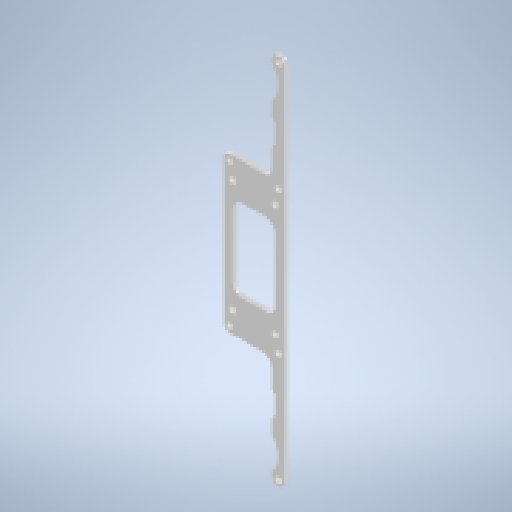
# Autodesk Inventor part: new_ude
Saved by Autodesk Inventor 2024 (Build 280153000, 153)
## iProperties
Created: 2023-12-16
Part Number: new_ude
Material: アルミニウム 2014-T4
Document SubType Name: Modeling
Designer: right
Density: 2.8 g/cm^3
Appearance: サテン
Mass: 3.58939 g
Surface Area: 23.5034 cm^2
Volume: 1.28192 cm^3
Author: right
Autodesk Inventor part; units mm, degrees
ref_plane "YZ Plane" through (0, 0, 0) normal (1, 0, 0) x (0, 1, 0)
ref_plane "XZ Plane" through (0, 0, 0) normal (0, 1, 0) x (-1, 0, 0)
ref_plane "XY Plane" through (0, 0, 0) normal (0, 0, 1) x (1, 0, 0)
sketch "スケッチ1" plane through (0, 0, 0) normal (0, 0, 1) x (1, 0, 0)
  circle A0 centre (-5.2771, -42.7168) radius 0.85 projected
  circle A1 centre (-21.2771, -42.7168) radius 0.85 projected
  circle A2 centre (-5.2771, -6.7168) radius 0.85 projected
  circle A3 centre (-13.2771, -13.2168) radius 8 projected
  line L0 (-3.2771, -4.7168) -> (-7.2771, -4.7168)
  line L1 (-7.2771, -4.7168) -> (-7.2771, -44.7168)
  line L2 (-7.2771, -44.7168) -> (-3.2771, -44.7168)
  line L3 (-3.2771, -44.7168) -> (-3.2771, -4.7168)
  line L4 (-3.2771, -44.7168) -> (-23.2771, -44.7168)
  line L5 (-23.2771, -44.7168) -> (-23.2771, -40.7168)
  line L6 (-23.2771, -40.7168) -> (-3.2771, -40.7168)
  line L7 (-3.2771, -40.7168) -> (-3.2771, -44.7168)
  circle A4 centre (-5.2771, -6.7168) radius 2
  circle A5 centre (-21.2771, -42.7168) radius 2
  circle A6 centre (-5.2771, -6.7168) radius 1.1
  circle A7 centre (-5.2771, -42.7168) radius 1.1
  circle A8 centre (-21.2771, -42.7168) radius 1.1
  line L8 (-5.2771, -66.2168) -> (-21.2771, -66.2168) construction
  circle A9 centre (-5.2771, -89.7168) radius 0.85
  circle A10 centre (-21.2771, -89.7168) radius 0.85
  circle A11 centre (-5.2771, -125.7168) radius 0.85
  circle A12 centre (-13.2771, -119.2168) radius 8
  line L9 (-3.2771, -127.7168) -> (-7.2771, -127.7168)
  line L10 (-7.2771, -127.7168) -> (-7.2771, -87.7168)
  line L11 (-7.2771, -87.7168) -> (-3.2771, -87.7168)
  line L12 (-3.2771, -87.7168) -> (-3.2771, -127.7168)
  line L13 (-3.2771, -87.7168) -> (-23.2771, -87.7168)
  line L14 (-23.2771, -87.7168) -> (-23.2771, -91.7168)
  line L15 (-23.2771, -91.7168) -> (-3.2771, -91.7168)
  line L16 (-3.2771, -91.7168) -> (-3.2771, -87.7168)
  circle A13 centre (-5.2771, -125.7168) radius 2
  circle A14 centre (-21.2771, -89.7168) radius 2
  circle A15 centre (-5.2771, -125.7168) radius 1.1
  circle A16 centre (-5.2771, -89.7168) radius 1.1
  circle A17 centre (-21.2771, -89.7168) radius 1.1
  line L17 (-3.2771, -44.7168) -> (-3.2771, -87.7168)
  line L18 (-23.2771, -44.7168) -> (-23.2771, -87.7168)
  line L19 (-6.4151, -24.526) -> (-6.4151, -30.526)
  line L20 (-6.2865, -24.2474) -> (-6.2865, -30.6046)
  line L21 (-6.2865, -30.6046) -> (-10.1437, -30.6046)
  line L22 (-10.1437, -24.2474) -> (-6.2865, -24.2474)
  line L23 (-6.4151, -107.9075) -> (-6.4151, -101.9075)
  line L24 (-6.2865, -108.1861) -> (-6.2865, -101.8289)
  line L25 (-6.2865, -101.8289) -> (-10.1437, -101.8289)
  line L26 (-10.1437, -108.1861) -> (-6.2865, -108.1861)
  line L27 (7.0429, 25.428) -> (7.0429, 23.728)
  point P0 (0, 0)
  point P1 (-3.2771, -42.7168)
  point P2 (-5.2771, -4.7168)
  point P3 (-13.2771, -44.7168)
  point P4 (-13.2771, -66.2168)
  point P5 (-3.2771, -89.7168)
  point P6 (-5.2771, -127.7168)
  point P7 (-13.2771, -87.7168)
  point P8 (-7.2771, -6.7168)
  point P9 (-7.2771, -7.9253)
  point P10 (-7.2771, -18.5083)
  point P11 (-7.2771, -40.7168)
  point P12 (-21.2771, -40.7168)
  point P13 (-23.2771, -42.7168)
  point P14 (-23.2771, -89.7168)
  point P15 (-21.2771, -91.7168)
  point P16 (-7.2771, -91.7168)
  point P17 (-7.2771, -113.9253)
  point P18 (-7.2771, -124.5083)
  point P19 (-7.2771, -125.7168)
  point P20 (-3.2771, -125.7168)
  point P21 (-3.2771, -6.7168)
  point P22 (-7.2771, -24.2474)
  point P23 (-7.2771, -30.6046)
  point P24 (-7.2771, -101.8289)
  point P25 (-7.2771, -108.1861)
  point P26 (7.0429, 24.578)
  dimension "d0" = 4
  dimension "d1" = 4
  dimension "d2" = 2.2
  dimension "d3" = 2.2
  dimension "d4" = 2.2
  dimension "d11" = 53
  constraints: 56 end point, 25 symmetric about line, 14 centre point, 10 coincident, 5 horizontal, 5 midpoint, 5 vertical, 4 parallel, 4 tangent, 2 perpendicular, 2 vertical alignment, 1 horizontal alignment, 17 other
  measures "d0" distance between parallel lines of L3 L1
  measures "d1" diameter of A5
  measures "d2" diameter of A6
  measures "d3" diameter of A7
  measures "d4" diameter of A8
  measures "d11" distance from line of A3.centre L8
extrude "押し出し1" add sketch "スケッチ1" along normal blind 1.5 contours A3 L1 A4 L3 L6 L21 L20 L22 | A4 | L3 L2 L1 L6 | L1 L4 A5 L6 | L17 L11 L13 L18 L4 L2 | A5 | L12 L15 L10 L11 | L4 L5 A5 | L10 L15 A14 L13 | L12 A13 L10 A12 L26 L24 L25 L15 | A14 L14 L13 | A14 | A13
fillet "フィレット1" radius 2 4 edges at (-7.2771, -108.1861, 0.75) (-7.2771, -101.8289, 0.75) (-7.2771, -24.2474, 0.75) (-7.2771, -30.6046, 0.75)
fillet "フィレット2" radius 2 4 edges at (-7.2771, -18.5083, 0.75) (-7.2771, -7.9253, 0.75) (-7.2771, -124.5083, 0.75) (-7.2771, -113.9253, 0.75)
fillet "フィレット3" radius 3 2 edges at (-7.2771, -91.7168, 0.75) (-7.2771, -40.7168, 0.75)
sketch "スケッチ2" plane through (0, 0, 1.5) normal (0, 0, 1) x (1, 0, 0)
  circle A0 centre (-6.2771, -47.7168) radius 1.1
  line L0 (-3.2771, -125.7168) -> (-3.2771, -6.7168) projected
  circle A1 centre (-5.2771, -42.7168) radius 1.1 projected
  circle A2 centre (-20.2771, -47.7168) radius 1.1
  line L1 (-23.2771, -42.7168) -> (-23.2771, -89.7168) projected
  line L2 (-3.2771, -66.2168) -> (-23.2771, -66.2168) construction
  circle A3 centre (-6.2771, -84.7168) radius 1.1
  circle A4 centre (-20.2771, -84.7168) radius 1.1
  line L3 (-20.2771, -52.7168) -> (-6.2771, -52.7168)
  line L4 (-6.2771, -52.7168) -> (-6.2771, -79.7168)
  line L5 (-6.2771, -79.7168) -> (-20.2771, -79.7168)
  line L6 (-20.2771, -79.7168) -> (-20.2771, -52.7168)
  line L7 (-20.2771, -52.7168) -> (-6.2771, -79.7168) construction
  line L8 (-6.2771, -52.7168) -> (-20.2771, -79.7168) construction
  point P0 (0, 0)
  point P1 (-13.2771, -66.2168)
  dimension "d12" = 2.2
  dimension "d13" = 3
  dimension "d14" = 5
  dimension "d15" = 2.2
  dimension "d16" = 3
  dimension "d17" = 5
  dimension "d18" = 3
  constraints: 14 end point, 5 midpoint, 4 centre point, 2 parallel, 2 symmetric about line, 1 horizontal, 1 horizontal alignment, 1 perpendicular, 2 other
  measures "d12" diameter of A0
  measures "d13" distance from line of L0 A0.centre
  measures "d14" vertical distance of A1.centre A0.centre
  measures "d15" diameter of A2
  measures "d16" distance from line of L1 A2.centre
  measures "d17" distance from line of A0.centre L3
  measures "d18" distance between parallel lines of L0 L4
extrude "押し出し2" cut sketch "スケッチ2" against normal blind 1.5 contours A0 | A2 | A3 | A4 | L3 L4 L5 L6
fillet "フィレット4" radius 3 4 edges at (-20.2771, -52.7168, 0.75) (-6.2771, -52.7168, 0.75) (-20.2771, -79.7168, 0.75) (-6.2771, -79.7168, 0.75)
equation "\"d16\" = d13"
